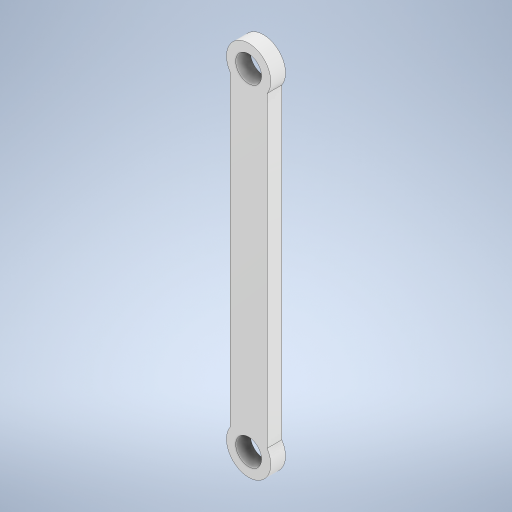
# Autodesk Inventor part: legparts_03(seven)
Saved by Autodesk Inventor 2024.3 (Build 283343000, 343)
## iProperties
Created: 2024-10-20
Part Number: legparts_03(seven)
Material: ABS プラスチック
Document SubType Name: Modeling
Designer: 佐藤智貴
Density: 1.06 g/cm^3
Appearance: 滑らか - 白
Mass: 39.825 g
Surface Area: 123.708 cm^2
Volume: 37.5708 cm^3
Author: 佐藤智貴
Autodesk Inventor part; units mm, degrees
ref_plane "YZ Plane" through (0, 0, 0) normal (1, 0, 0) x (0, 1, 0)
ref_plane "XZ Plane" through (0, 0, 0) normal (0, 1, 0) x (-1, 0, 0)
ref_plane "XY Plane" through (0, 0, 0) normal (0, 0, 1) x (1, 0, 0)
sketch "スケッチ1" plane through (0, 0, 0) normal (0, 0, 1) x (1, 0, 0)
  circle A0 centre (0, 0) radius 7
  circle A1 centre (0, 0) radius 12
  line L0 (-5, 4.899) -> (5, 4.899)
  line L1 (5, 4.899) -> (5, -188.5584)
  line L2 (5, -188.5584) -> (-5, -188.5584)
  line L3 (-5, -188.5584) -> (-5, 4.899)
  circle A2 centre (0, -180) radius 7
  circle A3 centre (0, -180) radius 12
  line L4 (10, -193.5584) -> (10, 9.899)
  line L5 (10, 9.899) -> (-10, 9.899)
  line L6 (-10, 9.899) -> (-10, -193.5584)
  line L7 (-10, -193.5584) -> (10, -193.5584)
  point P0 (5, -10.9087)
  point P1 (-5, -10.9087)
  point P2 (-8, 8.9443)
  point P3 (12, 0)
  point P4 (-5, -169.0913)
  point P5 (5, -169.0913)
  point P6 (0, -188.5584)
  point P7 (10, -173.3668)
  point P8 (10, -6.6332)
  point P9 (-10, -6.6332)
  point P10 (-10, -173.3668)
  dimension "d0" = 14
  dimension "d1" = 24
  dimension "d3" = 10
  dimension "d16" = 14
  dimension "d17" = 24
  dimension "d22" = 180
  dimension "d23" = 5
  dimension "d24" = 0
  dimension "d25" = 5
  constraints: 16 end point, 4 parallel, 3 centre point, 2 perpendicular, 2 point on circle, 1 coincident, 1 horizontal, 1 midpoint, 6 other
  measures "d1" diameter of A1
  measures "d3" distance of L0.start L0.end
  measures "d16" diameter of A2
  measures "d17" diameter of A3
  measures "d22" distance of A2.centre A1.centre
  measures "d23" distance from line of point (0, 0) L1
  measures "d24" horizontal distance of point (0, -188.558) A2.centre
  measures "d25" distance between parallel lines of L3 L6
extrude "押し出し1" add sketch "スケッチ1" along normal blind 8 contours A0 L3 A1 L6 L5 L4 L1 | L1 A1 L3 A0 | L1 A3 L3 A1 | A1 L4 A3 L1 | L3 A3 L6 A1 | L4 A1 | A3 L4 L6 L3 A2 L2 L1 | L1 A2 L3 A3 | A1 L6 | A3 L4 | L6 A3 | L5 A1 | L1 L2 L3 A2
equation "\"d23\" = 0.5 * d3"
